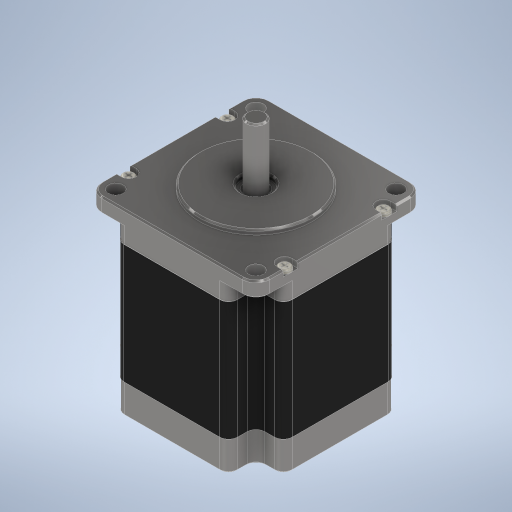
# Autodesk Inventor part: Motor
Saved by Autodesk Inventor 2023 (Build 270158000, 158)
## iProperties
Created: 2023-10-12
Part Number: Motor
Material: Stainless Steel, 440C
Document SubType Name: Sheet Metal
Designer: Mateus Quintino
Density: 7.75 g/cm^3
Sheet Metal Rule: Default_mm
Appearance: Glossy - Black
Author: Mateus Quintino
Autodesk Inventor part; units mm, degrees
(part 1 of 2)
ref_plane "YZ Plane" through (0, 0, 0) normal (1, 0, 0) x (0, 1, 0)
ref_plane "XZ Plane" through (0, 0, 0) normal (0, 1, 0) x (-1, 0, 0)
sketch "Sketch1" plane through (0, 0, 0) normal (0, 1, 0) x (-1, 0, 0)
  line L0 (28.2, 19) -> (28.2, -19)
  line L1 (28.2, -19) -> (19, -19)
  line L2 (19, -19) -> (19, -28.2)
  line L3 (19, -28.2) -> (-19, -28.2)
  line L4 (-19, -28.2) -> (-19, -19)
  line L5 (-19, -19) -> (-28.2, -19)
  line L6 (-28.2, -19) -> (-28.2, 19)
  line L7 (-28.2, 19) -> (-19, 19)
  line L8 (-19, 19) -> (-19, 28.2)
  line L9 (-19, 28.2) -> (19, 28.2)
  line L10 (19, 28.2) -> (19, 19)
  line L11 (19, 19) -> (28.2, 19)
  point P0 (0, 0)
  dimension "d7" = 56.4
  dimension "d9" = 28.2
  dimension "d10" = 28.2
  dimension "d12" = 38
  constraints: 24 end point, 9 equal length, 4 horizontal, 4 perpendicular, 3 parallel, 1 vertical
  measures "d7" distance between parallel lines of L9 L3
  measures "d9" distance from line of L0 point (0, 0)
  measures "d10" distance from line of point (0, 0) L3
  measures "d12" distance between parallel lines of L4 L2
extrude "Extrusion1" add sketch "Sketch1" along normal blind 10
sketch "Sketch2" plane through (0, 10, 0) normal (0, 1, 0) x (1, 0, 0)
  line L0 (-19, -19) -> (-19, -28.2) projected
  line L1 (-19, -28.2) -> (19, -28.2) projected
  line L2 (19, -28.2) -> (19, -19) projected
  line L3 (19, -19) -> (28.2, -19) projected
  line L4 (28.2, -19) -> (28.2, 19) projected
  line L5 (28.2, 19) -> (19, 19) projected
  line L6 (19, 19) -> (19, 28.2) projected
  line L7 (19, 28.2) -> (-19, 28.2) projected
  line L8 (-19, 28.2) -> (-19, 19) projected
  line L9 (-19, 19) -> (-28.2, 19) projected
  line L10 (-28.2, 19) -> (-28.2, -19) projected
  line L11 (-28.2, -19) -> (-19, -19) projected
  line L12 (-19.1, 28.3) -> (19.1, 28.3)
  line L13 (19.1, 28.3) -> (19.1, 19.1)
  line L14 (19.1, 19.1) -> (28.3, 19.1)
  line L15 (28.3, 19.1) -> (28.3, -19.1)
  line L16 (28.3, -19.1) -> (19.1, -19.1)
  line L17 (19.1, -19.1) -> (19.1, -28.3)
  line L18 (19.1, -28.3) -> (-19.1, -28.3)
  line L19 (-19.1, -28.3) -> (-19.1, -19.1)
  line L20 (-19.1, -19.1) -> (-28.3, -19.1)
  line L21 (-28.3, -19.1) -> (-28.3, 19.1)
  line L22 (-28.3, 19.1) -> (-19.1, 19.1)
  line L23 (-19.1, 19.1) -> (-19.1, 28.3)
  point P0 (0, 0)
  dimension "d15" = 0.1
  constraints: 24 end point, 11 other
  measures "d15" distance between parallel lines of L7 L12
extrude "Extrusion2" add sketch "Sketch2" along normal blind 40 contours L11 L10 L9 L8 L7 L6 L5 L4 L3 L2 L1 L0 | L12 L13 L14 L15 L16 L17 L18 L19 L20 L21 L22 L23
sketch "Sketch3" plane through (0, 50, 0) normal (0, 1, 0) x (1, 0, 0)
  line L0 (-19, -19) -> (-19, -28.2) projected
  line L1 (-28.2, -19) -> (-19, -19) projected
  line L2 (-28.2, 19) -> (-28.2, -19) projected
  line L3 (-19, 19) -> (-28.2, 19) projected
  line L4 (-19, 28.2) -> (-19, 19) projected
  line L5 (19, 28.2) -> (-19, 28.2) projected
  line L6 (19, 19) -> (19, 28.2) projected
  line L7 (28.2, 19) -> (19, 19) projected
  line L8 (28.2, -19) -> (28.2, 19) projected
  line L9 (19, -19) -> (28.2, -19) projected
  line L10 (19, -28.2) -> (19, -19) projected
  line L11 (-19, -28.2) -> (19, -28.2) projected
  point P0 (0, 0)
extrude "Extrusion3" add sketch "Sketch3" along normal blind 5
sketch "Sketch4" plane through (0, 55, 0) normal (0, 1, 0) x (1, 0, 0)
  line L0 (-28.2, -28.2) -> (28.2, -28.2)
  line L1 (28.2, -28.2) -> (28.2, 28.2)
  line L2 (28.2, 28.2) -> (-28.2, 28.2)
  line L3 (-28.2, 28.2) -> (-28.2, -28.2)
  line L4 (-28.2, -28.2) -> (28.2, 28.2) construction
  line L5 (28.2, -28.2) -> (-28.2, 28.2) construction
  line L6 (19, 28.2) -> (-19, 28.2) projected
  line L7 (-19, -28.2) -> (19, -28.2) projected
  point P0 (0, 0)
  dimension "d20" = 56.4
  dimension "d21" = 56.4
  constraints: 12 end point, 2 midpoint, 2 parallel, 2 perpendicular, 1 horizontal
  measures "d20" distance between parallel lines of L6 L7
  measures "d21" distance of L0.end L1.end
extrude "Extrusion4" add sketch "Sketch4" along normal blind 5
sketch "Sketch5" plane through (0, 60, 0) normal (0, 1, 0) x (1, 0, 0)
  circle A0 centre (0, 0) radius 19
  dimension "d24" = 38
  constraints: 1 centre point, 1 coincident
  measures "d24" diameter of A0
extrude "Extrusion5" add sketch "Sketch5" along normal blind 1.6
sketch "Sketch6" plane through (0, 61.6, 0) normal (0, 1, 0) x (1, 0, 0)
  circle A0 centre (0, 0) radius 5
  dimension "d27" = 10
  constraints: 1 centre point, 1 coincident
  measures "d27" diameter of A0
extrude "Extrusion6" cut sketch "Sketch6" against normal blind 1.6
sketch "Sketch7" plane through (0, 60, 0) normal (0, 1, 0) x (1, 0, 0)
  circle A0 centre (0, 0) radius 3.325
  dimension "d30" = 6.65
  constraints: 1 centre point, 1 coincident
  measures "d30" diameter of A0
extrude "Extrusion7" cut sketch "Sketch7" against normal blind 5
sketch "Sketch8" plane through (0, 55, 0) normal (0, 1, 0) x (1, 0, 0)
  circle A0 centre (0, 0) radius 3.175
  dimension "d33" = 6.35
  constraints: 1 centre point, 1 coincident
  measures "d33" diameter of A0
extrude "Extrusion8" add sketch "Sketch8" along normal blind 26
fillet "Fillet1" radius 3 36 edges at (19, 52.5, 19) (19.1, 30, 19.1) (19, 5, 19) (19, 5, 28.2) (19.1, 30, 28.3) (19, 52.5, 28.2) (28.2, 52.5, 19) (28.3, 30, 19.1) (28.2, 5, 19) (-19, 52.5, 28.2) (-19.1, 30, 28.3) (-19, 5, 28.2) (-19.1, 30, 19.1) (-19, 52.5, 19) (-28.2, 52.5, 19) (-28.3, 30, 19.1) (-28.2, 5, 19) (-19, 5, 19) (-28.2, 5, -19) (-28.3, 30, -19.1) (-28.2, 52.5, -19) (-19, 52.5, -19) (-19.1, 30, -19.1) (-19, 5, -19) (-19, 5, -28.2) (-19.1, 30, -28.3) (-19, 52.5, -28.2) (19, 52.5, -28.2) (19.1, 30, -28.3) (19, 5, -28.2) (19, 5, -19) (28.2, 5, -19) (28.3, 30, -19.1) (19.1, 30, -19.1) (19, 52.5, -19) (28.2, 52.5, -19)
sketch "Sketch9" plane through (0, 60, 0) normal (0, 1, 0) x (1, 0, 0)
  line L0 (-23.55, 23.55) -> (23.55, 23.55)
  line L1 (23.55, 23.55) -> (23.55, -23.55)
  line L2 (23.55, -23.55) -> (-23.55, -23.55)
  line L3 (-23.55, -23.55) -> (-23.55, 23.55)
  circle A0 centre (0, 0) radius 3.175 projected
  line L4 (-23.55, 23.55) -> (23.55, -23.55) construction
  line L5 (23.55, 23.55) -> (-23.55, -23.55) construction
  circle A1 centre (23.55, 23.55) radius 2.5
  circle A2 centre (-23.55, 23.55) radius 2.5
  circle A3 centre (-23.55, -23.55) radius 2.5
  circle A4 centre (23.55, -23.55) radius 2.5
  dimension "d40" = 47.1
  dimension "d41" = 5
  constraints: 12 end point, 4 centre point, 4 coincident, 3 equal radius, 2 midpoint, 2 parallel, 2 perpendicular, 1 horizontal
  measures "d40" distance of L0.start L0.end
  measures "d41" diameter of A1
extrude "Extrusion9" cut sketch "Sketch9" against normal up to surface (5 mm away) contours L3 A2 L0 | L0 A2 L3 | A1 L1 L0 | L0 L1 A1 | A3 L2 L3 | L3 L2 A3 | A4 L2 L1 | L1 L2 A4
fillet "Fillet2" radius 4.65 4 edges at (28.2, 57.5, -28.2) (28.2, 57.5, 28.2) (-28.2, 57.5, -28.2) (-28.2, 57.5, 28.2)
chamfer "Chamfer1" distance 0.5 angle 45 1 edges at (-3.175, 81, 0)
chamfer "Chamfer2" distance 0.5 angle 45 3 edges at (-19, 61.6, 0) (-3.325, 60, 0) (-5, 61.6, 0)
chamfer "Chamfer4" distance 0.5 angle 45 12 edges at (28.2, 55, -19.775) (26.838, 55, -26.838) (19.775, 55, -28.2) (-19.775, 55, -28.2) (-26.838, 55, -26.838) (-28.2, 55, -19.775) (28.2, 55, 19.775) (26.838, 55, 26.838) (19.775, 55, 28.2) (-26.838, 55, 26.838) (-19.775, 55, 28.2) (-28.2, 55, 19.775)
sketch "Sketch10" plane through (0, 60, 0) normal (0, 1, 0) x (1, 0, 0)
  line L0 (19.1, -25.3) -> (19.1, -22.1) projected
  line L1 (-19.1, -22.1) -> (-19.1, -25.3) projected
  line L2 (-25.3, -19.1) -> (-22.1, -19.1) projected
  line L3 (-22.1, 19.1) -> (-25.3, 19.1) projected
  line L4 (-19.1, 25.3) -> (-19.1, 22.1) projected
  line L5 (19.1, 22.1) -> (19.1, 25.3) projected
  line L6 (22.1, -19.1) -> (25.3, -19.1) projected
  line L7 (-26.2, -19.1) -> (-28.2, -19.1)
  line L8 (-23.7, -16.6) -> (-23.7, -16.6)
  line L9 (-26.2, -14.1) -> (-28.2, -14.1)
  arc A0 (-26.2, -19.1) -> (-23.7, -16.6) centre (-26.2, -16.6) ccw
  arc A1 (-23.7, -16.6) -> (-26.2, -14.1) centre (-26.2, -16.6) ccw
  line L10 (-28.2, 23.55) -> (-28.2, -23.55) projected
  line L11 (-28.2, -14.1) -> (-28.2, -19.1)
  line L12 (-28.2, 0) -> (28.2, 0)
  line L13 (28.2, -23.55) -> (28.2, 23.55) projected
  line L14 (-25.3, 19.1) -> (-22.1, 19.1)
  line L15 (-26.2, 19.1) -> (-28.2, 19.1)
  line L16 (-26.2, 14.1) -> (-28.2, 14.1)
  arc A2 (-23.7, 16.6) -> (-26.2, 19.1) centre (-26.2, 16.6) ccw
  arc A3 (-26.2, 14.1) -> (-23.7, 16.6) centre (-26.2, 16.6) ccw
  line L17 (-28.2, 14.1) -> (-28.2, 19.1)
  line L18 (0, -28.3) -> (0, 28.3)
  line L19 (25.3, -19.1) -> (22.1, -19.1)
  line L20 (22.1, 19.1) -> (25.3, 19.1)
  line L21 (26.2, -19.1) -> (28.2, -19.1)
  line L22 (23.7, -16.6) -> (23.7, -16.6)
  line L23 (26.2, -14.1) -> (28.2, -14.1)
  arc A4 (23.7, -16.6) -> (26.2, -19.1) centre (26.2, -16.6) ccw
  arc A5 (26.2, -14.1) -> (23.7, -16.6) centre (26.2, -16.6) ccw
  line L24 (28.2, -14.1) -> (28.2, -19.1)
  line L25 (25.3, 19.1) -> (22.1, 19.1)
  arc A6 (23.7, 16.6) -> (26.2, 14.1) centre (26.2, 16.6) ccw
  line L26 (26.2, 14.1) -> (28.2, 14.1)
  arc A7 (26.2, 19.1) -> (23.7, 16.6) centre (26.2, 16.6) ccw
  line L27 (28.2, 14.1) -> (28.2, 19.1)
  line L28 (26.2, 19.1) -> (28.2, 19.1)
  point P0 (0, 0)
  point P1 (-23.7, -19.1)
  point P2 (-23.7, -14.1)
  point P3 (-23.7, 19.1)
  point P4 (-23.7, 14.1)
  point P5 (23.7, -19.1)
  point P6 (23.7, -14.1)
  point P7 (23.7, 14.1)
  point P8 (23.7, 19.1)
  dimension "d57" = 5
  dimension "d58" = 2.5
  constraints: 40 end point, 30 symmetric about line, 16 point on circle, 14 point on line, 8 centre point, 4 tangent, 3 midpoint, 3 perpendicular, 2 vertical, 1 collinear, 1 concentric, 1 horizontal, 6 other
  measures "d57" distance of point (-23.7, -19.1) point (-23.7, -14.1)
  measures "d58" radius of A0
extrude "Extrusion10" cut sketch "Sketch10" against normal blind 2
sketch "Sketch11" plane through (0, 58, 0) normal (0, 1, 0) x (1, 0, 0)
  arc A0 (-26.2, -19.1) -> (-26.2, -14.1) centre (-26.2, -16.6) ccw projected
  circle A1 centre (-26.2, -16.6) radius 2
  arc A2 (-26.2, 14.1) -> (-26.2, 19.1) centre (-26.2, 16.6) ccw projected
  circle A3 centre (-26.2, 16.6) radius 2
  arc A4 (26.2, 19.1) -> (26.2, 14.1) centre (26.2, 16.6) ccw projected
  circle A5 centre (26.2, 16.6) radius 2
  arc A6 (26.2, -14.1) -> (26.2, -19.1) centre (26.2, -16.6) ccw projected
  circle A7 centre (26.2, -16.6) radius 2
  point P0 (0, 0)
  dimension "d62" = 4
  constraints: 4 centre point, 4 coincident, 3 equal radius
  measures "d62" diameter of A1
extrude "Extrusion11" add sketch "Sketch11" along normal blind 1.25
fillet "Fillet3" radius 0.6 4 edges at (24.2, 59.25, 16.6) (24.2, 59.25, -16.6) (-28.2, 59.25, -16.6) (-28.2, 59.25, 16.6)
sketch "Sketch12" plane through (-26.2, 59.25, 16.6) normal (0, 1, 0) x (1, 0, 0)
  line L0 (-0.2, -1.25) -> (-0.2, -0.2)
  line L1 (-0.2, -0.2) -> (-1.25, -0.2)
  line L2 (-1.25, -0.2) -> (-1.25, 0.2)
  line L3 (-1.25, 0.2) -> (-0.2, 0.2)
  line L4 (-0.2, 0.2) -> (-0.2, 1.25)
  line L5 (-0.2, 1.25) -> (0.2, 1.25)
  line L6 (0.2, 1.25) -> (0.2, 0.2)
  line L7 (0.2, 0.2) -> (1.25, 0.2)
  line L8 (1.25, 0.2) -> (1.25, -0.2)
  line L9 (1.25, -0.2) -> (0.2, -0.2)
  line L10 (0.2, -0.2) -> (0.2, -1.25)
  line L11 (0.2, -1.25) -> (-0.2, -1.25)
  circle A0 centre (0, 0) radius 1.4 projected
  line L12 (26.2, 16.6) -> (-2, 16.6)
  line L13 (-2, 0.6) -> (-2, 32.6) projected
  circle A1 centre (26.2, 16.6) radius 3.175 projected
  line L14 (26.2, 16.6) -> (26.2, -11.6)
  line L15 (10.2, -11.6) -> (42.2, -11.6) projected
  line L16 (-0.2, 34.45) -> (-0.2, 33.4)
  line L17 (-0.2, 33.4) -> (-1.25, 33.4)
  line L18 (-1.25, 33.4) -> (-1.25, 33)
  line L19 (-1.25, 33) -> (-0.2, 33)
  line L20 (-0.2, 33) -> (-0.2, 31.95)
  line L21 (-0.2, 31.95) -> (0.2, 31.95)
  line L22 (0.2, 31.95) -> (0.2, 33)
  line L23 (0.2, 33) -> (1.25, 33)
  line L24 (1.25, 33) -> (1.25, 33.4)
  line L25 (1.25, 33.4) -> (0.2, 33.4)
  line L26 (0.2, 33.4) -> (0.2, 34.45)
  line L27 (0.2, 34.45) -> (-0.2, 34.45)
  circle A2 centre (0, 33.2) radius 1.4
  line L28 (52.6, -1.25) -> (52.6, -0.2)
  line L29 (52.6, -0.2) -> (53.65, -0.2)
  line L30 (53.65, -0.2) -> (53.65, 0.2)
  line L31 (53.65, 0.2) -> (52.6, 0.2)
  line L32 (52.6, 0.2) -> (52.6, 1.25)
  line L33 (52.6, 1.25) -> (52.2, 1.25)
  line L34 (52.2, 1.25) -> (52.2, 0.2)
  line L35 (52.2, 0.2) -> (51.15, 0.2)
  line L36 (51.15, 0.2) -> (51.15, -0.2)
  line L37 (51.15, -0.2) -> (52.2, -0.2)
  line L38 (52.2, -0.2) -> (52.2, -1.25)
  line L39 (52.2, -1.25) -> (52.6, -1.25)
  circle A3 centre (52.4, 0) radius 1.4
  line L40 (54.4, 0.6) -> (54.4, 32.6)
  line L41 (52.6, 33) -> (52.6, 31.95)
  line L42 (52.2, 31.95) -> (52.2, 33)
  line L43 (53.65, 33) -> (52.6, 33)
  line L44 (52.2, 33) -> (51.15, 33)
  line L45 (53.65, 33.4) -> (53.65, 33)
  line L46 (52.6, 33.4) -> (53.65, 33.4)
  line L47 (51.15, 33.4) -> (52.2, 33.4)
  line L48 (51.15, 33) -> (51.15, 33.4)
  line L49 (52.6, 34.45) -> (52.6, 33.4)
  line L50 (52.2, 34.45) -> (52.6, 34.45)
  line L51 (52.2, 33.4) -> (52.2, 34.45)
  circle A4 centre (52.4, 33.2) radius 1.4
  line L52 (52.6, 31.95) -> (52.2, 31.95)
  point P0 (54.4, 16.6)
  dimension "d66" = 2.5
  dimension "d67" = 2.5
  dimension "d68" = 0.4
  dimension "d69" = 1.25
  dimension "d70" = 1.25
  constraints: 102 end point, 42 symmetric about line, 24 point on line, 8 perpendicular, 5 equal length, 3 centre point, 2 midpoint, 1 vertical, 3 other
  measures "d66" distance between parallel lines of L11 L5
  measures "d67" distance between parallel lines of L2 L8
  measures "d68" distance of L4.end L5.end
  measures "d69" distance from line of A0.centre L2
  measures "d70" distance from line of A0.centre L11
extrude "Extrusion12" cut sketch "Sketch12" against normal blind 1 contours L0 L1 L2 L3 L4 L5 L6 L7 L8 L9 L10 L11 | L27 L26 L25 L24 L23 L22 L21 L20 L19 L18 L17 L16 | L39 L38 L37 L36 L35 L34 L33 L32 L31 L30 L29 L28 | L41 L52 L42 L44 L48 L47 L51 L50 L49 L46 L45 L43
fillet "Fillet4" radius 0.3 16 edges at (26, 58.75, 16.4) (26.4, 58.75, 16.4) (26, 58.75, 16.8) (26.4, 58.75, 16.8) (26, 58.75, -16.8) (26, 58.75, -16.4) (26.4, 58.75, -16.8) (26.4, 58.75, -16.4) (-26, 58.75, -16.4) (-26.4, 58.75, -16.4) (-26, 58.75, -16.8) (-26.4, 58.75, -16.8) (-26.4, 58.75, 16.8) (-26.4, 58.75, 16.4) (-26, 58.75, 16.4) (-26, 58.75, 16.8)
sketch "Sketch13" plane through (28.3, 10, 16.1) normal (1, 0, 0) x (0, 0, -1)
  arc A0 (-12.2, 40) -> (-12.125, 39.8701) centre (-12.05, 40) ccw
  arc A1 (-12.125, 39.6103) -> (-12.125, 39.8701) centre (-12.2, 39.7402) ccw
  arc A2 (-12.125, 39.6103) -> (-12.2, 39.4804) centre (-12.05, 39.4804) ccw
  line L0 (-12.2, 40) -> (-9.2, 40) projected
  line L1 (-9.2, 0) -> (-9.2, 40) projected
  arc A3 (-12.2, 39.4804) -> (-12.125, 39.3505) centre (-12.05, 39.4804) ccw
  arc A4 (-12.125, 39.0907) -> (-12.125, 39.3505) centre (-12.2, 39.2206) ccw
  arc A5 (-12.125, 39.0907) -> (-12.2, 38.9608) centre (-12.05, 38.9608) ccw
  arc A6 (-12.2, 38.9608) -> (-12.125, 38.8309) centre (-12.05, 38.9608) ccw
  arc A7 (-12.125, 38.5711) -> (-12.125, 38.8309) centre (-12.2, 38.701) ccw
  arc A8 (-12.125, 38.5711) -> (-12.2, 38.4412) centre (-12.05, 38.4412) ccw
  arc A9 (-12.2, 38.4412) -> (-12.125, 38.3113) centre (-12.05, 38.4412) ccw
  arc A10 (-12.125, 38.0514) -> (-12.125, 38.3113) centre (-12.2, 38.1813) ccw
  arc A11 (-12.125, 38.0514) -> (-12.2, 37.9215) centre (-12.05, 37.9215) ccw
  arc A12 (-12.2, 37.9215) -> (-12.125, 37.7916) centre (-12.05, 37.9215) ccw
  arc A13 (-12.125, 37.5318) -> (-12.125, 37.7916) centre (-12.2, 37.6617) ccw
  arc A14 (-12.125, 37.5318) -> (-12.2, 37.4019) centre (-12.05, 37.4019) ccw
  arc A15 (-12.2, 37.4019) -> (-12.125, 37.272) centre (-12.05, 37.4019) ccw
  arc A16 (-12.125, 37.0122) -> (-12.125, 37.272) centre (-12.2, 37.1421) ccw
  arc A17 (-12.125, 37.0122) -> (-12.2, 36.8823) centre (-12.05, 36.8823) ccw
  arc A18 (-12.2, 36.8823) -> (-12.125, 36.7524) centre (-12.05, 36.8823) ccw
  arc A19 (-12.125, 36.4926) -> (-12.125, 36.7524) centre (-12.2, 36.6225) ccw
  arc A20 (-12.125, 36.4926) -> (-12.2, 36.3627) centre (-12.05, 36.3627) ccw
  arc A21 (-12.2, 36.3627) -> (-12.125, 36.2328) centre (-12.05, 36.3627) ccw
  arc A22 (-12.125, 35.973) -> (-12.125, 36.2328) centre (-12.2, 36.1029) ccw
  arc A23 (-12.125, 35.973) -> (-12.2, 35.8431) centre (-12.05, 35.8431) ccw
  arc A24 (-12.2, 35.8431) -> (-12.125, 35.7132) centre (-12.05, 35.8431) ccw
  arc A25 (-12.125, 35.4534) -> (-12.125, 35.7132) centre (-12.2, 35.5833) ccw
  arc A26 (-12.125, 35.4534) -> (-12.2, 35.3235) centre (-12.05, 35.3235) ccw
  arc A27 (-12.2, 35.3235) -> (-12.125, 35.1936) centre (-12.05, 35.3235) ccw
  arc A28 (-12.125, 34.9338) -> (-12.125, 35.1936) centre (-12.2, 35.0637) ccw
  arc A29 (-12.125, 34.9338) -> (-12.2, 34.8038) centre (-12.05, 34.8038) ccw
  arc A30 (-12.2, 34.8038) -> (-12.125, 34.6739) centre (-12.05, 34.8038) ccw
  arc A31 (-12.125, 34.4141) -> (-12.125, 34.6739) centre (-12.2, 34.544) ccw
  arc A32 (-12.125, 34.4141) -> (-12.2, 34.2842) centre (-12.05, 34.2842) ccw
  arc A33 (-12.2, 34.2842) -> (-12.125, 34.1543) centre (-12.05, 34.2842) ccw
  arc A34 (-12.125, 33.8945) -> (-12.125, 34.1543) centre (-12.2, 34.0244) ccw
  arc A35 (-12.125, 33.8945) -> (-12.2, 33.7646) centre (-12.05, 33.7646) ccw
  arc A36 (-12.2, 33.7646) -> (-12.125, 33.6347) centre (-12.05, 33.7646) ccw
  arc A37 (-12.125, 33.3749) -> (-12.125, 33.6347) centre (-12.2, 33.5048) ccw
  arc A38 (-12.125, 33.3749) -> (-12.2, 33.245) centre (-12.05, 33.245) ccw
  arc A39 (-12.2, 33.245) -> (-12.125, 33.1151) centre (-12.05, 33.245) ccw
  arc A40 (-12.125, 32.8553) -> (-12.125, 33.1151) centre (-12.2, 32.9852) ccw
  arc A41 (-12.125, 32.8553) -> (-12.2, 32.7254) centre (-12.05, 32.7254) ccw
  arc A42 (-12.2, 32.7254) -> (-12.125, 32.5955) centre (-12.05, 32.7254) ccw
  arc A43 (-12.125, 32.3357) -> (-12.125, 32.5955) centre (-12.2, 32.4656) ccw
  arc A44 (-12.125, 32.3357) -> (-12.2, 32.2058) centre (-12.05, 32.2058) ccw
  arc A45 (-12.2, 32.2058) -> (-12.125, 32.0759) centre (-12.05, 32.2058) ccw
  arc A46 (-12.125, 31.8161) -> (-12.125, 32.0759) centre (-12.2, 31.946) ccw
  arc A47 (-12.125, 31.8161) -> (-12.2, 31.6862) centre (-12.05, 31.6862) ccw
  arc A48 (-12.2, 31.6862) -> (-12.125, 31.5563) centre (-12.05, 31.6862) ccw
  arc A49 (-12.125, 31.2964) -> (-12.125, 31.5563) centre (-12.2, 31.4263) ccw
  arc A50 (-12.125, 31.2964) -> (-12.2, 31.1665) centre (-12.05, 31.1665) ccw
  arc A51 (-12.2, 31.1665) -> (-12.125, 31.0366) centre (-12.05, 31.1665) ccw
  arc A52 (-12.125, 30.7768) -> (-12.125, 31.0366) centre (-12.2, 30.9067) ccw
  arc A53 (-12.125, 30.7768) -> (-12.2, 30.6469) centre (-12.05, 30.6469) ccw
  arc A54 (-12.2, 30.6469) -> (-12.125, 30.517) centre (-12.05, 30.6469) ccw
  arc A55 (-12.125, 30.2572) -> (-12.125, 30.517) centre (-12.2, 30.3871) ccw
  arc A56 (-12.125, 30.2572) -> (-12.2, 30.1273) centre (-12.05, 30.1273) ccw
  arc A57 (-12.2, 30.1273) -> (-12.125, 29.9974) centre (-12.05, 30.1273) ccw
  arc A58 (-12.125, 29.7376) -> (-12.125, 29.9974) centre (-12.2, 29.8675) ccw
  arc A59 (-12.125, 29.7376) -> (-12.2, 29.6077) centre (-12.05, 29.6077) ccw
  arc A60 (-12.2, 29.6077) -> (-12.125, 29.4778) centre (-12.05, 29.6077) ccw
  arc A61 (-12.125, 29.218) -> (-12.125, 29.4778) centre (-12.2, 29.3479) ccw
  arc A62 (-12.125, 29.218) -> (-12.2, 29.0881) centre (-12.05, 29.0881) ccw
  arc A63 (-12.2, 29.0881) -> (-12.125, 28.9582) centre (-12.05, 29.0881) ccw
  arc A64 (-12.125, 28.6984) -> (-12.125, 28.9582) centre (-12.2, 28.8283) ccw
  arc A65 (-12.125, 28.6984) -> (-12.2, 28.5685) centre (-12.05, 28.5685) ccw
  arc A66 (-12.2, 28.5685) -> (-12.125, 28.4386) centre (-12.05, 28.5685) ccw
  arc A67 (-12.125, 28.1788) -> (-12.125, 28.4386) centre (-12.2, 28.3087) ccw
  arc A68 (-12.125, 28.1788) -> (-12.2, 28.0488) centre (-12.05, 28.0488) ccw
  arc A69 (-12.2, 28.0488) -> (-12.125, 27.9189) centre (-12.05, 28.0488) ccw
  arc A70 (-12.125, 27.6591) -> (-12.125, 27.9189) centre (-12.2, 27.789) ccw
  arc A71 (-12.125, 27.6591) -> (-12.2, 27.5292) centre (-12.05, 27.5292) ccw
  arc A72 (-12.2, 27.5292) -> (-12.125, 27.3993) centre (-12.05, 27.5292) ccw
  arc A73 (-12.125, 27.1395) -> (-12.125, 27.3993) centre (-12.2, 27.2694) ccw
  arc A74 (-12.125, 27.1395) -> (-12.2, 27.0096) centre (-12.05, 27.0096) ccw
  arc A75 (-12.2, 27.0096) -> (-12.125, 26.8797) centre (-12.05, 27.0096) ccw
  arc A76 (-12.125, 26.6199) -> (-12.125, 26.8797) centre (-12.2, 26.7498) ccw
  arc A77 (-12.125, 26.6199) -> (-12.2, 26.49) centre (-12.05, 26.49) ccw
  arc A78 (-12.2, 26.49) -> (-12.125, 26.3601) centre (-12.05, 26.49) ccw
  arc A79 (-12.125, 26.1003) -> (-12.125, 26.3601) centre (-12.2, 26.2302) ccw
  arc A80 (-12.125, 26.1003) -> (-12.2, 25.9704) centre (-12.05, 25.9704) ccw
  arc A81 (-12.2, 25.9704) -> (-12.125, 25.8405) centre (-12.05, 25.9704) ccw
  arc A82 (-12.125, 25.5807) -> (-12.125, 25.8405) centre (-12.2, 25.7106) ccw
  arc A83 (-12.125, 25.5807) -> (-12.2, 25.4508) centre (-12.05, 25.4508) ccw
  arc A84 (-12.2, 25.4508) -> (-12.125, 25.3209) centre (-12.05, 25.4508) ccw
  arc A85 (-12.125, 25.0611) -> (-12.125, 25.3209) centre (-12.2, 25.191) ccw
  arc A86 (-12.125, 25.0611) -> (-12.2, 24.9312) centre (-12.05, 24.9312) ccw
  arc A87 (-12.2, 24.9312) -> (-12.125, 24.8013) centre (-12.05, 24.9312) ccw
  arc A88 (-12.125, 24.5414) -> (-12.125, 24.8013) centre (-12.2, 24.6714) ccw
  arc A89 (-12.125, 24.5414) -> (-12.2, 24.4115) centre (-12.05, 24.4115) ccw
  arc A90 (-12.2, 24.4115) -> (-12.125, 24.2816) centre (-12.05, 24.4115) ccw
  arc A91 (-12.125, 24.0218) -> (-12.125, 24.2816) centre (-12.2, 24.1517) ccw
  arc A92 (-12.125, 24.0218) -> (-12.2, 23.8919) centre (-12.05, 23.8919) ccw
  arc A93 (-12.2, 23.8919) -> (-12.125, 23.762) centre (-12.05, 23.8919) ccw
  arc A94 (-12.125, 23.5022) -> (-12.125, 23.762) centre (-12.2, 23.6321) ccw
  arc A95 (-12.125, 23.5022) -> (-12.2, 23.3723) centre (-12.05, 23.3723) ccw
  arc A96 (-12.2, 23.3723) -> (-12.125, 23.2424) centre (-12.05, 23.3723) ccw
  arc A97 (-12.125, 22.9826) -> (-12.125, 23.2424) centre (-12.2, 23.1125) ccw
  arc A98 (-12.125, 22.9826) -> (-12.2, 22.8527) centre (-12.05, 22.8527) ccw
  arc A99 (-12.2, 22.8527) -> (-12.125, 22.7228) centre (-12.05, 22.8527) ccw
  arc A100 (-12.125, 22.463) -> (-12.125, 22.7228) centre (-12.2, 22.5929) ccw
  arc A101 (-12.125, 22.463) -> (-12.2, 22.3331) centre (-12.05, 22.3331) ccw
  arc A102 (-12.2, 22.3331) -> (-12.125, 22.2032) centre (-12.05, 22.3331) ccw
  arc A103 (-12.125, 21.9434) -> (-12.125, 22.2032) centre (-12.2, 22.0733) ccw
  arc A104 (-12.125, 21.9434) -> (-12.2, 21.8135) centre (-12.05, 21.8135) ccw
  arc A105 (-12.2, 21.8135) -> (-12.125, 21.6836) centre (-12.05, 21.8135) ccw
  arc A106 (-12.125, 21.4238) -> (-12.125, 21.6836) centre (-12.2, 21.5537) ccw
  arc A107 (-12.125, 21.4238) -> (-12.2, 21.2939) centre (-12.05, 21.2939) ccw
  arc A108 (-12.2, 21.2939) -> (-12.125, 21.1639) centre (-12.05, 21.2939) ccw
  arc A109 (-12.125, 20.9041) -> (-12.125, 21.1639) centre (-12.2, 21.034) ccw
  arc A110 (-12.125, 20.9041) -> (-12.2, 20.7742) centre (-12.05, 20.7742) ccw
  arc A111 (-12.2, 20.7742) -> (-12.125, 20.6443) centre (-12.05, 20.7742) ccw
  arc A112 (-12.125, 20.3845) -> (-12.125, 20.6443) centre (-12.2, 20.5144) ccw
  arc A113 (-12.125, 20.3845) -> (-12.2, 20.2546) centre (-12.05, 20.2546) ccw
  arc A114 (-12.2, 20.2546) -> (-12.125, 20.1247) centre (-12.05, 20.2546) ccw
  arc A115 (-12.125, 19.8649) -> (-12.125, 20.1247) centre (-12.2, 19.9948) ccw
  arc A116 (-12.125, 19.8649) -> (-12.2, 19.735) centre (-12.05, 19.735) ccw
  arc A117 (-12.2, 19.735) -> (-12.125, 19.6051) centre (-12.05, 19.735) ccw
  arc A118 (-12.125, 19.3453) -> (-12.125, 19.6051) centre (-12.2, 19.4752) ccw
  arc A119 (-12.125, 19.3453) -> (-12.2, 19.2154) centre (-12.05, 19.2154) ccw
  arc A120 (-12.2, 19.2154) -> (-12.125, 19.0855) centre (-12.05, 19.2154) ccw
  arc A121 (-12.125, 18.8257) -> (-12.125, 19.0855) centre (-12.2, 18.9556) ccw
  arc A122 (-12.125, 18.8257) -> (-12.2, 18.6958) centre (-12.05, 18.6958) ccw
  arc A123 (-12.2, 18.6958) -> (-12.125, 18.5659) centre (-12.05, 18.6958) ccw
  arc A124 (-12.125, 18.3061) -> (-12.125, 18.5659) centre (-12.2, 18.436) ccw
  arc A125 (-12.125, 18.3061) -> (-12.2, 18.1762) centre (-12.05, 18.1762) ccw
  arc A126 (-12.2, 18.1762) -> (-12.125, 18.0463) centre (-12.05, 18.1762) ccw
  arc A127 (-12.125, 17.7864) -> (-12.125, 18.0463) centre (-12.2, 17.9164) ccw
  arc A128 (-12.125, 17.7864) -> (-12.2, 17.6565) centre (-12.05, 17.6565) ccw
  arc A129 (-12.2, 17.6565) -> (-12.125, 17.5266) centre (-12.05, 17.6565) ccw
  arc A130 (-12.125, 17.2668) -> (-12.125, 17.5266) centre (-12.2, 17.3967) ccw
  arc A131 (-12.125, 17.2668) -> (-12.2, 17.1369) centre (-12.05, 17.1369) ccw
  arc A132 (-12.2, 17.1369) -> (-12.125, 17.007) centre (-12.05, 17.1369) ccw
  arc A133 (-12.125, 16.7472) -> (-12.125, 17.007) centre (-12.2, 16.8771) ccw
  arc A134 (-12.125, 16.7472) -> (-12.2, 16.6173) centre (-12.05, 16.6173) ccw
  arc A135 (-12.2, 16.6173) -> (-12.125, 16.4874) centre (-12.05, 16.6173) ccw
  arc A136 (-12.125, 16.2276) -> (-12.125, 16.4874) centre (-12.2, 16.3575) ccw
  arc A137 (-12.125, 16.2276) -> (-12.2, 16.0977) centre (-12.05, 16.0977) ccw
  arc A138 (-12.2, 16.0977) -> (-12.125, 15.9678) centre (-12.05, 16.0977) ccw
  arc A139 (-12.125, 15.708) -> (-12.125, 15.9678) centre (-12.2, 15.8379) ccw
  arc A140 (-12.125, 15.708) -> (-12.2, 15.5781) centre (-12.05, 15.5781) ccw
  arc A141 (-12.2, 15.5781) -> (-12.125, 15.4482) centre (-12.05, 15.5781) ccw
  arc A142 (-12.125, 15.1884) -> (-12.125, 15.4482) centre (-12.2, 15.3183) ccw
  arc A143 (-12.125, 15.1884) -> (-12.2, 15.0585) centre (-12.05, 15.0585) ccw
  arc A144 (-12.2, 15.0585) -> (-12.125, 14.9286) centre (-12.05, 15.0585) ccw
  arc A145 (-12.125, 14.6688) -> (-12.125, 14.9286) centre (-12.2, 14.7987) ccw
  arc A146 (-12.125, 14.6688) -> (-12.2, 14.5389) centre (-12.05, 14.5389) ccw
  arc A147 (-12.2, 14.5389) -> (-12.125, 14.4089) centre (-12.05, 14.5389) ccw
  arc A148 (-12.125, 14.1491) -> (-12.125, 14.4089) centre (-12.2, 14.279) ccw
  arc A149 (-12.125, 14.1491) -> (-12.2, 14.0192) centre (-12.05, 14.0192) ccw
  arc A150 (-12.2, 14.0192) -> (-12.125, 13.8893) centre (-12.05, 14.0192) ccw
  arc A151 (-12.125, 13.6295) -> (-12.125, 13.8893) centre (-12.2, 13.7594) ccw
  arc A152 (-12.125, 13.6295) -> (-12.2, 13.4996) centre (-12.05, 13.4996) ccw
  arc A153 (-12.2, 13.4996) -> (-12.125, 13.3697) centre (-12.05, 13.4996) ccw
  arc A154 (-12.125, 13.1099) -> (-12.125, 13.3697) centre (-12.2, 13.2398) ccw
  arc A155 (-12.125, 13.1099) -> (-12.2, 12.98) centre (-12.05, 12.98) ccw
  arc A156 (-12.2, 12.98) -> (-12.125, 12.8501) centre (-12.05, 12.98) ccw
  arc A157 (-12.125, 12.5903) -> (-12.125, 12.8501) centre (-12.2, 12.7202) ccw
  arc A158 (-12.125, 12.5903) -> (-12.2, 12.4604) centre (-12.05, 12.4604) ccw
  arc A159 (-12.2, 12.4604) -> (-12.125, 12.3305) centre (-12.05, 12.4604) ccw
  arc A160 (-12.125, 12.0707) -> (-12.125, 12.3305) centre (-12.2, 12.2006) ccw
  arc A161 (-12.125, 12.0707) -> (-12.2, 11.9408) centre (-12.05, 11.9408) ccw
  arc A162 (-12.2, 11.9408) -> (-12.125, 11.8109) centre (-12.05, 11.9408) ccw
  arc A163 (-12.125, 11.5511) -> (-12.125, 11.8109) centre (-12.2, 11.681) ccw
  arc A164 (-12.125, 11.5511) -> (-12.2, 11.4212) centre (-12.05, 11.4212) ccw
  arc A165 (-12.2, 11.4212) -> (-12.125, 11.2913) centre (-12.05, 11.4212) ccw
  arc A166 (-12.125, 11.0315) -> (-12.125, 11.2913) centre (-12.2, 11.1614) ccw
  arc A167 (-12.125, 11.0315) -> (-12.2, 10.9015) centre (-12.05, 10.9015) ccw
  arc A168 (-12.2, 10.9015) -> (-12.125, 10.7716) centre (-12.05, 10.9015) ccw
  arc A169 (-12.125, 10.5118) -> (-12.125, 10.7716) centre (-12.2, 10.6417) ccw
  arc A170 (-12.125, 10.5118) -> (-12.2, 10.3819) centre (-12.05, 10.3819) ccw
  arc A171 (-12.2, 10.3819) -> (-12.125, 10.252) centre (-12.05, 10.3819) ccw
  arc A172 (-12.125, 9.9922) -> (-12.125, 10.252) centre (-12.2, 10.1221) ccw
  arc A173 (-12.125, 9.9922) -> (-12.2, 9.8623) centre (-12.05, 9.8623) ccw
  arc A174 (-12.2, 9.8623) -> (-12.125, 9.7324) centre (-12.05, 9.8623) ccw
  arc A175 (-12.125, 9.4726) -> (-12.125, 9.7324) centre (-12.2, 9.6025) ccw
  arc A176 (-12.125, 9.4726) -> (-12.2, 9.3427) centre (-12.05, 9.3427) ccw
  arc A177 (-12.2, 9.3427) -> (-12.125, 9.2128) centre (-12.05, 9.3427) ccw
  arc A178 (-12.125, 8.953) -> (-12.125, 9.2128) centre (-12.2, 9.0829) ccw
  arc A179 (-12.125, 8.953) -> (-12.2, 8.8231) centre (-12.05, 8.8231) ccw
  arc A180 (-12.2, 8.8231) -> (-12.125, 8.6932) centre (-12.05, 8.8231) ccw
  arc A181 (-12.125, 8.4334) -> (-12.125, 8.6932) centre (-12.2, 8.5633) ccw
  arc A182 (-12.125, 8.4334) -> (-12.2, 8.3035) centre (-12.05, 8.3035) ccw
  arc A183 (-12.2, 8.3035) -> (-12.125, 8.1736) centre (-12.05, 8.3035) ccw
  arc A184 (-12.125, 7.9138) -> (-12.125, 8.1736) centre (-12.2, 8.0437) ccw
  arc A185 (-12.125, 7.9138) -> (-12.2, 7.7839) centre (-12.05, 7.7839) ccw
  arc A186 (-12.2, 7.7839) -> (-12.125, 7.654) centre (-12.05, 7.7839) ccw
  arc A187 (-12.125, 7.3941) -> (-12.125, 7.654) centre (-12.2, 7.524) ccw
  arc A188 (-12.125, 7.3941) -> (-12.2, 7.2642) centre (-12.05, 7.2642) ccw
  arc A189 (-12.2, 7.2642) -> (-12.125, 7.1343) centre (-12.05, 7.2642) ccw
  arc A190 (-12.125, 6.8745) -> (-12.125, 7.1343) centre (-12.2, 7.0044) ccw
  arc A191 (-12.125, 6.8745) -> (-12.2, 6.7446) centre (-12.05, 6.7446) ccw
  arc A192 (-12.2, 6.7446) -> (-12.125, 6.6147) centre (-12.05, 6.7446) ccw
  arc A193 (-12.125, 6.3549) -> (-12.125, 6.6147) centre (-12.2, 6.4848) ccw
  arc A194 (-12.125, 6.3549) -> (-12.2, 6.225) centre (-12.05, 6.225) ccw
  arc A195 (-12.2, 6.225) -> (-12.125, 6.0951) centre (-12.05, 6.225) ccw
  arc A196 (-12.125, 5.8353) -> (-12.125, 6.0951) centre (-12.2, 5.9652) ccw
  arc A197 (-12.125, 5.8353) -> (-12.2, 5.7054) centre (-12.05, 5.7054) ccw
  arc A198 (-12.2, 5.7054) -> (-12.125, 5.5755) centre (-12.05, 5.7054) ccw
  arc A199 (-12.125, 5.3157) -> (-12.125, 5.5755) centre (-12.2, 5.4456) ccw
  arc A200 (-12.125, 5.3157) -> (-12.2, 5.1858) centre (-12.05, 5.1858) ccw
  arc A201 (-12.2, 5.1858) -> (-12.125, 5.0559) centre (-12.05, 5.1858) ccw
  arc A202 (-12.125, 4.7961) -> (-12.125, 5.0559) centre (-12.2, 4.926) ccw
  arc A203 (-12.125, 4.7961) -> (-12.2, 4.6662) centre (-12.05, 4.6662) ccw
  arc A204 (-12.2, 4.6662) -> (-12.125, 4.5363) centre (-12.05, 4.6662) ccw
  arc A205 (-12.125, 4.2765) -> (-12.125, 4.5363) centre (-12.2, 4.4064) ccw
  arc A206 (-12.125, 4.2765) -> (-12.2, 4.1465) centre (-12.05, 4.1465) ccw
  arc A207 (-12.2, 4.1465) -> (-12.125, 4.0166) centre (-12.05, 4.1465) ccw
  arc A208 (-12.125, 3.7568) -> (-12.125, 4.0166) centre (-12.2, 3.8867) ccw
  arc A209 (-12.125, 3.7568) -> (-12.2, 3.6269) centre (-12.05, 3.6269) ccw
  arc A210 (-12.2, 3.6269) -> (-12.125, 3.497) centre (-12.05, 3.6269) ccw
  arc A211 (-12.125, 3.2372) -> (-12.125, 3.497) centre (-12.2, 3.3671) ccw
  arc A212 (-12.125, 3.2372) -> (-12.2, 3.1073) centre (-12.05, 3.1073) ccw
  arc A213 (-12.2, 3.1073) -> (-12.125, 2.9774) centre (-12.05, 3.1073) ccw
  arc A214 (-12.125, 2.7176) -> (-12.125, 2.9774) centre (-12.2, 2.8475) ccw
  arc A215 (-12.125, 2.7176) -> (-12.2, 2.5877) centre (-12.05, 2.5877) ccw
  arc A216 (-12.2, 2.5877) -> (-12.125, 2.4578) centre (-12.05, 2.5877) ccw
  arc A217 (-12.125, 2.198) -> (-12.125, 2.4578) centre (-12.2, 2.3279) ccw
  arc A218 (-12.125, 2.198) -> (-12.2, 2.0681) centre (-12.05, 2.0681) ccw
  arc A219 (-12.2, 2.0681) -> (-12.125, 1.9382) centre (-12.05, 2.0681) ccw
  arc A220 (-12.125, 1.6784) -> (-12.125, 1.9382) centre (-12.2, 1.8083) ccw
  arc A221 (-12.125, 1.6784) -> (-12.2, 1.5485) centre (-12.05, 1.5485) ccw
  arc A222 (-12.2, 1.5485) -> (-12.125, 1.4186) centre (-12.05, 1.5485) ccw
  arc A223 (-12.125, 1.1588) -> (-12.125, 1.4186) centre (-12.2, 1.2887) ccw
  arc A224 (-12.125, 1.1588) -> (-12.2, 1.0289) centre (-12.05, 1.0289) ccw
  arc A225 (-12.2, 1.0289) -> (-12.125, 0.899) centre (-12.05, 1.0289) ccw
  arc A226 (-12.125, 0.6391) -> (-12.125, 0.899) centre (-12.2, 0.769) ccw
  arc A227 (-12.125, 0.6391) -> (-12.2, 0.5092) centre (-12.05, 0.5092) ccw
  arc A228 (-12.2, 0.5092) -> (-12.125, 0.3793) centre (-12.05, 0.5092) ccw
  arc A229 (-12.125, 0.1195) -> (-12.125, 0.3793) centre (-12.2, 0.2494) ccw
  arc A230 (-12.125, 0.1195) -> (-12.2, -0.0104) centre (-12.05, -0.0104) ccw
  line L2 (-12.2, -0.0104) -> (-12.6895, -0.0104)
  line L3 (-12.6895, -0.0104) -> (-12.6895, 40)
  line L4 (-12.6895, 40) -> (-12.2, 40)
  point P0 (16.1, -10)
  dimension "d75" = 0
  dimension "d76" = 0.15
  dimension "d77" = 0.5196
  dimension "d80" = 0.5196
  constraints: 462 point on circle, 231 centre point, 6 end point, 4 equal radius, 1 horizontal, 1 perpendicular, 1 point on line, 1 vertical, 760 other
  measures "d75" distance from line of L0 A0.centre
  measures "d76" radius of A0
  measures "d77" distance of L0.start A2.end
  measures "d80" distance of A0.centre A3.centre
ref_plane "Work Plane1" through (16.1, 10, 28.3) normal (1, 0, 0) x (0, -1, 0)
sketch "Sketch14" plane through (16.1, 10, 28.3) normal (1, 0, 0) x (0, -1, 0)
  line L0 (0.0104, -0.4895) -> (-40, -0.4895) projected
  line L1 (0.0104, 0) -> (0.0104, -0.4895) projected
  line L2 (-40, -0.4895) -> (-40, 0) projected
  arc A0 (-40, 0) -> (-39.8701, 0.075) centre (-40, 0.15) ccw
  arc A1 (-39.6103, 0.075) -> (-39.8701, 0.075) centre (-39.7402, 0) ccw
  arc A2 (-39.6103, 0.075) -> (-39.4804, 0) centre (-39.4804, 0.15) ccw
  arc A3 (-39.4804, 0) -> (-39.3505, 0.075) centre (-39.4804, 0.15) ccw
  arc A4 (-39.0907, 0.075) -> (-38.9608, 0) centre (-38.9608, 0.15) ccw
  arc A5 (-39.0907, 0.075) -> (-39.3505, 0.075) centre (-39.2206, 0) ccw
  arc A6 (-38.9608, 0) -> (-38.8309, 0.075) centre (-38.9608, 0.15) ccw
  arc A7 (-38.5711, 0.075) -> (-38.4412, 0) centre (-38.4412, 0.15) ccw
  arc A8 (-38.5711, 0.075) -> (-38.8309, 0.075) centre (-38.701, 0) ccw
  arc A9 (-38.4412, 0) -> (-38.3113, 0.075) centre (-38.4412, 0.15) ccw
  arc A10 (-38.0514, 0.075) -> (-37.9215, 0) centre (-37.9215, 0.15) ccw
  arc A11 (-38.0514, 0.075) -> (-38.3113, 0.075) centre (-38.1813, 0) ccw
  arc A12 (-37.9215, 0) -> (-37.7916, 0.075) centre (-37.9215, 0.15) ccw
  arc A13 (-37.5318, 0.075) -> (-37.4019, 0) centre (-37.4019, 0.15) ccw
  arc A14 (-37.5318, 0.075) -> (-37.7916, 0.075) centre (-37.6617, 0) ccw
  arc A15 (-37.4019, 0) -> (-37.272, 0.075) centre (-37.4019, 0.15) ccw
  arc A16 (-37.0122, 0.075) -> (-36.8823, 0) centre (-36.8823, 0.15) ccw
  arc A17 (-37.0122, 0.075) -> (-37.272, 0.075) centre (-37.1421, 0) ccw
  arc A18 (-36.8823, 0) -> (-36.7524, 0.075) centre (-36.8823, 0.15) ccw
  arc A19 (-36.4926, 0.075) -> (-36.3627, 0) centre (-36.3627, 0.15) ccw
  arc A20 (-36.4926, 0.075) -> (-36.7524, 0.075) centre (-36.6225, 0) ccw
  arc A21 (-36.3627, 0) -> (-36.2328, 0.075) centre (-36.3627, 0.15) ccw
  arc A22 (-35.973, 0.075) -> (-35.8431, 0) centre (-35.8431, 0.15) ccw
  arc A23 (-35.973, 0.075) -> (-36.2328, 0.075) centre (-36.1029, 0) ccw
  arc A24 (-35.8431, 0) -> (-35.7132, 0.075) centre (-35.8431, 0.15) ccw
  arc A25 (-35.4534, 0.075) -> (-35.3235, 0) centre (-35.3235, 0.15) ccw
  arc A26 (-35.4534, 0.075) -> (-35.7132, 0.075) centre (-35.5833, 0) ccw
  arc A27 (-35.3235, 0) -> (-35.1936, 0.075) centre (-35.3235, 0.15) ccw
  arc A28 (-34.9338, 0.075) -> (-34.8038, 0) centre (-34.8038, 0.15) ccw
  arc A29 (-34.9338, 0.075) -> (-35.1936, 0.075) centre (-35.0637, 0) ccw
  arc A30 (-34.8038, 0) -> (-34.6739, 0.075) centre (-34.8038, 0.15) ccw
  arc A31 (-34.4141, 0.075) -> (-34.2842, 0) centre (-34.2842, 0.15) ccw
  arc A32 (-34.4141, 0.075) -> (-34.6739, 0.075) centre (-34.544, 0) ccw
  arc A33 (-34.2842, 0) -> (-34.1543, 0.075) centre (-34.2842, 0.15) ccw
  arc A34 (-33.8945, 0.075) -> (-33.7646, 0) centre (-33.7646, 0.15) ccw
  arc A35 (-33.8945, 0.075) -> (-34.1543, 0.075) centre (-34.0244, 0) ccw
  arc A36 (-33.7646, 0) -> (-33.6347, 0.075) centre (-33.7646, 0.15) ccw
  arc A37 (-33.3749, 0.075) -> (-33.245, 0) centre (-33.245, 0.15) ccw
  arc A38 (-33.3749, 0.075) -> (-33.6347, 0.075) centre (-33.5048, 0) ccw
  arc A39 (-33.245, 0) -> (-33.1151, 0.075) centre (-33.245, 0.15) ccw
  arc A40 (-32.8553, 0.075) -> (-32.7254, 0) centre (-32.7254, 0.15) ccw
  arc A41 (-32.8553, 0.075) -> (-33.1151, 0.075) centre (-32.9852, 0) ccw
  arc A42 (-32.7254, 0) -> (-32.5955, 0.075) centre (-32.7254, 0.15) ccw
  arc A43 (-32.3357, 0.075) -> (-32.2058, 0) centre (-32.2058, 0.15) ccw
  arc A44 (-32.3357, 0.075) -> (-32.5955, 0.075) centre (-32.4656, 0) ccw
  arc A45 (-32.2058, 0) -> (-32.0759, 0.075) centre (-32.2058, 0.15) ccw
  arc A46 (-31.8161, 0.075) -> (-31.6862, 0) centre (-31.6862, 0.15) ccw
  arc A47 (-31.8161, 0.075) -> (-32.0759, 0.075) centre (-31.946, 0) ccw
  arc A48 (-31.6862, 0) -> (-31.5563, 0.075) centre (-31.6862, 0.15) ccw
  arc A49 (-31.2964, 0.075) -> (-31.1665, 0) centre (-31.1665, 0.15) ccw
  arc A50 (-31.2964, 0.075) -> (-31.5563, 0.075) centre (-31.4263, 0) ccw
  arc A51 (-31.1665, 0) -> (-31.0366, 0.075) centre (-31.1665, 0.15) ccw
  arc A52 (-30.7768, 0.075) -> (-30.6469, 0) centre (-30.6469, 0.15) ccw
  arc A53 (-30.7768, 0.075) -> (-31.0366, 0.075) centre (-30.9067, 0) ccw
  arc A54 (-30.6469, 0) -> (-30.517, 0.075) centre (-30.6469, 0.15) ccw
  arc A55 (-30.2572, 0.075) -> (-30.1273, 0) centre (-30.1273, 0.15) ccw
  arc A56 (-30.2572, 0.075) -> (-30.517, 0.075) centre (-30.3871, 0) ccw
  arc A57 (-30.1273, 0) -> (-29.9974, 0.075) centre (-30.1273, 0.15) ccw
  arc A58 (-29.7376, 0.075) -> (-29.6077, 0) centre (-29.6077, 0.15) ccw
  arc A59 (-29.7376, 0.075) -> (-29.9974, 0.075) centre (-29.8675, 0) ccw
  arc A60 (-29.6077, 0) -> (-29.4778, 0.075) centre (-29.6077, 0.15) ccw
  arc A61 (-29.218, 0.075) -> (-29.0881, 0) centre (-29.0881, 0.15) ccw
  arc A62 (-29.218, 0.075) -> (-29.4778, 0.075) centre (-29.3479, 0) ccw
  arc A63 (-29.0881, 0) -> (-28.9582, 0.075) centre (-29.0881, 0.15) ccw
  arc A64 (-28.6984, 0.075) -> (-28.5685, 0) centre (-28.5685, 0.15) ccw
  arc A65 (-28.6984, 0.075) -> (-28.9582, 0.075) centre (-28.8283, 0) ccw
  arc A66 (-28.5685, 0) -> (-28.4386, 0.075) centre (-28.5685, 0.15) ccw
  arc A67 (-28.1788, 0.075) -> (-28.0488, 0) centre (-28.0488, 0.15) ccw
  arc A68 (-28.1788, 0.075) -> (-28.4386, 0.075) centre (-28.3087, 0) ccw
  arc A69 (-28.0488, 0) -> (-27.9189, 0.075) centre (-28.0488, 0.15) ccw
  arc A70 (-27.6591, 0.075) -> (-27.5292, 0) centre (-27.5292, 0.15) ccw
  arc A71 (-27.6591, 0.075) -> (-27.9189, 0.075) centre (-27.789, 0) ccw
  arc A72 (-27.5292, 0) -> (-27.3993, 0.075) centre (-27.5292, 0.15) ccw
  arc A73 (-27.1395, 0.075) -> (-27.0096, 0) centre (-27.0096, 0.15) ccw
  arc A74 (-27.1395, 0.075) -> (-27.3993, 0.075) centre (-27.2694, 0) ccw
  arc A75 (-27.0096, 0) -> (-26.8797, 0.075) centre (-27.0096, 0.15) ccw
  arc A76 (-26.6199, 0.075) -> (-26.49, 0) centre (-26.49, 0.15) ccw
  arc A77 (-26.6199, 0.075) -> (-26.8797, 0.075) centre (-26.7498, 0) ccw
  arc A78 (-26.49, 0) -> (-26.3601, 0.075) centre (-26.49, 0.15) ccw
  arc A79 (-26.1003, 0.075) -> (-25.9704, 0) centre (-25.9704, 0.15) ccw
  arc A80 (-26.1003, 0.075) -> (-26.3601, 0.075) centre (-26.2302, 0) ccw
  arc A81 (-25.9704, 0) -> (-25.8405, 0.075) centre (-25.9704, 0.15) ccw
  arc A82 (-25.5807, 0.075) -> (-25.4508, 0) centre (-25.4508, 0.15) ccw
  arc A83 (-25.5807, 0.075) -> (-25.8405, 0.075) centre (-25.7106, 0) ccw
  arc A84 (-25.4508, 0) -> (-25.3209, 0.075) centre (-25.4508, 0.15) ccw
  arc A85 (-25.0611, 0.075) -> (-24.9312, 0) centre (-24.9312, 0.15) ccw
  arc A86 (-25.0611, 0.075) -> (-25.3209, 0.075) centre (-25.191, 0) ccw
  arc A87 (-24.9312, 0) -> (-24.8013, 0.075) centre (-24.9312, 0.15) ccw
  arc A88 (-24.5414, 0.075) -> (-24.4115, 0) centre (-24.4115, 0.15) ccw
  arc A89 (-24.5414, 0.075) -> (-24.8013, 0.075) centre (-24.6714, 0) ccw
  arc A90 (-24.4115, 0) -> (-24.2816, 0.075) centre (-24.4115, 0.15) ccw
  arc A91 (-24.0218, 0.075) -> (-23.8919, 0) centre (-23.8919, 0.15) ccw
  arc A92 (-24.0218, 0.075) -> (-24.2816, 0.075) centre (-24.1517, 0) ccw
  arc A93 (-23.8919, 0) -> (-23.762, 0.075) centre (-23.8919, 0.15) ccw
  arc A94 (-23.5022, 0.075) -> (-23.3723, 0) centre (-23.3723, 0.15) ccw
  arc A95 (-23.5022, 0.075) -> (-23.762, 0.075) centre (-23.6321, 0) ccw
  arc A96 (-23.3723, 0) -> (-23.2424, 0.075) centre (-23.3723, 0.15) ccw
  arc A97 (-22.9826, 0.075) -> (-22.8527, 0) centre (-22.8527, 0.15) ccw
  arc A98 (-22.9826, 0.075) -> (-23.2424, 0.075) centre (-23.1125, 0) ccw
  arc A99 (-22.8527, 0) -> (-22.7228, 0.075) centre (-22.8527, 0.15) ccw
  arc A100 (-22.463, 0.075) -> (-22.3331, 0) centre (-22.3331, 0.15) ccw
  arc A101 (-22.463, 0.075) -> (-22.7228, 0.075) centre (-22.5929, 0) ccw
  arc A102 (-22.3331, 0) -> (-22.2032, 0.075) centre (-22.3331, 0.15) ccw
  arc A103 (-21.9434, 0.075) -> (-21.8135, 0) centre (-21.8135, 0.15) ccw
  arc A104 (-21.9434, 0.075) -> (-22.2032, 0.075) centre (-22.0733, 0) ccw
  arc A105 (-21.8135, 0) -> (-21.6836, 0.075) centre (-21.8135, 0.15) ccw
  arc A106 (-21.4238, 0.075) -> (-21.2939, 0) centre (-21.2939, 0.15) ccw
  arc A107 (-21.4238, 0.075) -> (-21.6836, 0.075) centre (-21.5537, 0) ccw
  arc A108 (-21.2939, 0) -> (-21.1639, 0.075) centre (-21.2939, 0.15) ccw
  arc A109 (-20.9041, 0.075) -> (-20.7742, 0) centre (-20.7742, 0.15) ccw
  arc A110 (-20.9041, 0.075) -> (-21.1639, 0.075) centre (-21.034, 0) ccw
  arc A111 (-20.7742, 0) -> (-20.6443, 0.075) centre (-20.7742, 0.15) ccw
  arc A112 (-20.3845, 0.075) -> (-20.2546, 0) centre (-20.2546, 0.15) ccw
  arc A113 (-20.3845, 0.075) -> (-20.6443, 0.075) centre (-20.5144, 0) ccw
  arc A114 (-20.2546, 0) -> (-20.1247, 0.075) centre (-20.2546, 0.15) ccw
  arc A115 (-19.8649, 0.075) -> (-19.735, 0) centre (-19.735, 0.15) ccw
  arc A116 (-19.8649, 0.075) -> (-20.1247, 0.075) centre (-19.9948, 0) ccw
  arc A117 (-19.735, 0) -> (-19.6051, 0.075) centre (-19.735, 0.15) ccw
  arc A118 (-19.3453, 0.075) -> (-19.2154, 0) centre (-19.2154, 0.15) ccw
  arc A119 (-19.3453, 0.075) -> (-19.6051, 0.075) centre (-19.4752, 0) ccw
  arc A120 (-19.2154, 0) -> (-19.0855, 0.075) centre (-19.2154, 0.15) ccw
  arc A121 (-18.8257, 0.075) -> (-18.6958, 0) centre (-18.6958, 0.15) ccw
  arc A122 (-18.8257, 0.075) -> (-19.0855, 0.075) centre (-18.9556, 0) ccw
  arc A123 (-18.6958, 0) -> (-18.5659, 0.075) centre (-18.6958, 0.15) ccw
  arc A124 (-18.3061, 0.075) -> (-18.1762, 0) centre (-18.1762, 0.15) ccw
  arc A125 (-18.3061, 0.075) -> (-18.5659, 0.075) centre (-18.436, 0) ccw
  arc A126 (-18.1762, 0) -> (-18.0463, 0.075) centre (-18.1762, 0.15) ccw
  arc A127 (-17.7864, 0.075) -> (-17.6565, 0) centre (-17.6565, 0.15) ccw
  arc A128 (-17.7864, 0.075) -> (-18.0463, 0.075) centre (-17.9164, 0) ccw
  arc A129 (-17.6565, 0) -> (-17.5266, 0.075) centre (-17.6565, 0.15) ccw
  arc A130 (-17.2668, 0.075) -> (-17.1369, 0) centre (-17.1369, 0.15) ccw
  arc A131 (-17.2668, 0.075) -> (-17.5266, 0.075) centre (-17.3967, 0) ccw
  arc A132 (-17.1369, 0) -> (-17.007, 0.075) centre (-17.1369, 0.15) ccw
  arc A133 (-16.7472, 0.075) -> (-16.6173, 0) centre (-16.6173, 0.15) ccw
  arc A134 (-16.7472, 0.075) -> (-17.007, 0.075) centre (-16.8771, 0) ccw
  arc A135 (-16.6173, 0) -> (-16.4874, 0.075) centre (-16.6173, 0.15) ccw
  arc A136 (-16.2276, 0.075) -> (-16.0977, 0) centre (-16.0977, 0.15) ccw
  arc A137 (-16.2276, 0.075) -> (-16.4874, 0.075) centre (-16.3575, 0) ccw
  arc A138 (-16.0977, 0) -> (-15.9678, 0.075) centre (-16.0977, 0.15) ccw
  arc A139 (-15.708, 0.075) -> (-15.5781, 0) centre (-15.5781, 0.15) ccw
  arc A140 (-15.708, 0.075) -> (-15.9678, 0.075) centre (-15.8379, 0) ccw
  arc A141 (-15.5781, 0) -> (-15.4482, 0.075) centre (-15.5781, 0.15) ccw
  arc A142 (-15.1884, 0.075) -> (-15.0585, 0) centre (-15.0585, 0.15) ccw
  arc A143 (-15.1884, 0.075) -> (-15.4482, 0.075) centre (-15.3183, 0) ccw
  arc A144 (-15.0585, 0) -> (-14.9286, 0.075) centre (-15.0585, 0.15) ccw
  arc A145 (-14.6688, 0.075) -> (-14.5389, 0) centre (-14.5389, 0.15) ccw
  arc A146 (-14.6688, 0.075) -> (-14.9286, 0.075) centre (-14.7987, 0) ccw
  arc A147 (-14.5389, 0) -> (-14.4089, 0.075) centre (-14.5389, 0.15) ccw
  arc A148 (-14.1491, 0.075) -> (-14.0192, 0) centre (-14.0192, 0.15) ccw
  arc A149 (-14.1491, 0.075) -> (-14.4089, 0.075) centre (-14.279, 0) ccw
  arc A150 (-14.0192, 0) -> (-13.8893, 0.075) centre (-14.0192, 0.15) ccw
  arc A151 (-13.6295, 0.075) -> (-13.4996, 0) centre (-13.4996, 0.15) ccw
  arc A152 (-13.6295, 0.075) -> (-13.8893, 0.075) centre (-13.7594, 0) ccw
  arc A153 (-13.4996, 0) -> (-13.3697, 0.075) centre (-13.4996, 0.15) ccw
  arc A154 (-13.1099, 0.075) -> (-12.98, 0) centre (-12.98, 0.15) ccw
  arc A155 (-13.1099, 0.075) -> (-13.3697, 0.075) centre (-13.2398, 0) ccw
  arc A156 (-12.98, 0) -> (-12.8501, 0.075) centre (-12.98, 0.15) ccw
  arc A157 (-12.5903, 0.075) -> (-12.4604, 0) centre (-12.4604, 0.15) ccw
  arc A158 (-12.5903, 0.075) -> (-12.8501, 0.075) centre (-12.7202, 0) ccw
  arc A159 (-12.4604, 0) -> (-12.3305, 0.075) centre (-12.4604, 0.15) ccw
  arc A160 (-12.0707, 0.075) -> (-11.9408, 0) centre (-11.9408, 0.15) ccw
  arc A161 (-12.0707, 0.075) -> (-12.3305, 0.075) centre (-12.2006, 0) ccw
  arc A162 (-11.9408, 0) -> (-11.8109, 0.075) centre (-11.9408, 0.15) ccw
  arc A163 (-11.5511, 0.075) -> (-11.4212, 0) centre (-11.4212, 0.15) ccw
  arc A164 (-11.5511, 0.075) -> (-11.8109, 0.075) centre (-11.681, 0) ccw
  arc A165 (-11.4212, 0) -> (-11.2913, 0.075) centre (-11.4212, 0.15) ccw
  arc A166 (-11.0315, 0.075) -> (-10.9015, 0) centre (-10.9015, 0.15) ccw
  arc A167 (-11.0315, 0.075) -> (-11.2913, 0.075) centre (-11.1614, 0) ccw
  arc A168 (-10.9015, 0) -> (-10.7716, 0.075) centre (-10.9015, 0.15) ccw
  arc A169 (-10.5118, 0.075) -> (-10.3819, 0) centre (-10.3819, 0.15) ccw
  arc A170 (-10.5118, 0.075) -> (-10.7716, 0.075) centre (-10.6417, 0) ccw
  arc A171 (-10.3819, 0) -> (-10.252, 0.075) centre (-10.3819, 0.15) ccw
  arc A172 (-9.9922, 0.075) -> (-9.8623, 0) centre (-9.8623, 0.15) ccw
  arc A173 (-9.9922, 0.075) -> (-10.252, 0.075) centre (-10.1221, 0) ccw
  arc A174 (-9.8623, 0) -> (-9.7324, 0.075) centre (-9.8623, 0.15) ccw
  arc A175 (-9.4726, 0.075) -> (-9.3427, 0) centre (-9.3427, 0.15) ccw
  arc A176 (-9.4726, 0.075) -> (-9.7324, 0.075) centre (-9.6025, 0) ccw
  arc A177 (-9.3427, 0) -> (-9.2128, 0.075) centre (-9.3427, 0.15) ccw
  arc A178 (-8.953, 0.075) -> (-8.8231, 0) centre (-8.8231, 0.15) ccw
  arc A179 (-8.953, 0.075) -> (-9.2128, 0.075) centre (-9.0829, 0) ccw
  arc A180 (-8.8231, 0) -> (-8.6932, 0.075) centre (-8.8231, 0.15) ccw
  arc A181 (-8.4334, 0.075) -> (-8.3035, 0) centre (-8.3035, 0.15) ccw
  arc A182 (-8.4334, 0.075) -> (-8.6932, 0.075) centre (-8.5633, 0) ccw
  arc A183 (-8.3035, 0) -> (-8.1736, 0.075) centre (-8.3035, 0.15) ccw
  arc A184 (-7.9138, 0.075) -> (-7.7839, 0) centre (-7.7839, 0.15) ccw
  arc A185 (-7.9138, 0.075) -> (-8.1736, 0.075) centre (-8.0437, 0) ccw
  arc A186 (-7.7839, 0) -> (-7.654, 0.075) centre (-7.7839, 0.15) ccw
  arc A187 (-7.3941, 0.075) -> (-7.2642, 0) centre (-7.2642, 0.15) ccw
  arc A188 (-7.3941, 0.075) -> (-7.654, 0.075) centre (-7.524, 0) ccw
  arc A189 (-7.2642, 0) -> (-7.1343, 0.075) centre (-7.2642, 0.15) ccw
  arc A190 (-6.8745, 0.075) -> (-6.7446, 0) centre (-6.7446, 0.15) ccw
  arc A191 (-6.8745, 0.075) -> (-7.1343, 0.075) centre (-7.0044, 0) ccw
  arc A192 (-6.7446, 0) -> (-6.6147, 0.075) centre (-6.7446, 0.15) ccw
  arc A193 (-6.3549, 0.075) -> (-6.225, 0) centre (-6.225, 0.15) ccw
  arc A194 (-6.3549, 0.075) -> (-6.6147, 0.075) centre (-6.4848, 0) ccw
  arc A195 (-6.225, 0) -> (-6.0951, 0.075) centre (-6.225, 0.15) ccw
  arc A196 (-5.8353, 0.075) -> (-5.7054, 0) centre (-5.7054, 0.15) ccw
  arc A197 (-5.8353, 0.075) -> (-6.0951, 0.075) centre (-5.9652, 0) ccw
  arc A198 (-5.7054, 0) -> (-5.5755, 0.075) centre (-5.7054, 0.15) ccw
  arc A199 (-5.3157, 0.075) -> (-5.1858, 0) centre (-5.1858, 0.15) ccw
  arc A200 (-5.3157, 0.075) -> (-5.5755, 0.075) centre (-5.4456, 0) ccw
  arc A201 (-5.1858, 0) -> (-5.0559, 0.075) centre (-5.1858, 0.15) ccw
  arc A202 (-4.7961, 0.075) -> (-4.6662, 0) centre (-4.6662, 0.15) ccw
  arc A203 (-4.7961, 0.075) -> (-5.0559, 0.075) centre (-4.926, 0) ccw
  arc A204 (-4.6662, 0) -> (-4.5363, 0.075) centre (-4.6662, 0.15) ccw
  arc A205 (-4.2765, 0.075) -> (-4.1465, 0) centre (-4.1465, 0.15) ccw
  arc A206 (-4.2765, 0.075) -> (-4.5363, 0.075) centre (-4.4064, 0) ccw
  arc A207 (-4.1465, 0) -> (-4.0166, 0.075) centre (-4.1465, 0.15) ccw
  arc A208 (-3.7568, 0.075) -> (-3.6269, 0) centre (-3.6269, 0.15) ccw
  arc A209 (-3.7568, 0.075) -> (-4.0166, 0.075) centre (-3.8867, 0) ccw
  arc A210 (-3.6269, 0) -> (-3.497, 0.075) centre (-3.6269, 0.15) ccw
  arc A211 (-3.2372, 0.075) -> (-3.1073, 0) centre (-3.1073, 0.15) ccw
  arc A212 (-3.2372, 0.075) -> (-3.497, 0.075) centre (-3.3671, 0) ccw
  arc A213 (-3.1073, 0) -> (-2.9774, 0.075) centre (-3.1073, 0.15) ccw
  arc A214 (-2.7176, 0.075) -> (-2.5877, 0) centre (-2.5877, 0.15) ccw
  arc A215 (-2.7176, 0.075) -> (-2.9774, 0.075) centre (-2.8475, 0) ccw
  arc A216 (-2.5877, 0) -> (-2.4578, 0.075) centre (-2.5877, 0.15) ccw
  arc A217 (-2.198, 0.075) -> (-2.0681, 0) centre (-2.0681, 0.15) ccw
  arc A218 (-2.198, 0.075) -> (-2.4578, 0.075) centre (-2.3279, 0) ccw
  arc A219 (-2.0681, 0) -> (-1.9382, 0.075) centre (-2.0681, 0.15) ccw
  arc A220 (-1.6784, 0.075) -> (-1.5485, 0) centre (-1.5485, 0.15) ccw
  arc A221 (-1.6784, 0.075) -> (-1.9382, 0.075) centre (-1.8083, 0) ccw
  arc A222 (-1.5485, 0) -> (-1.4186, 0.075) centre (-1.5485, 0.15) ccw
  arc A223 (-1.1588, 0.075) -> (-1.0289, 0) centre (-1.0289, 0.15) ccw
  arc A224 (-1.1588, 0.075) -> (-1.4186, 0.075) centre (-1.2887, 0) ccw
  arc A225 (-1.0289, 0) -> (-0.899, 0.075) centre (-1.0289, 0.15) ccw
  arc A226 (-0.6391, 0.075) -> (-0.5092, 0) centre (-0.5092, 0.15) ccw
  arc A227 (-0.6391, 0.075) -> (-0.899, 0.075) centre (-0.769, 0) ccw